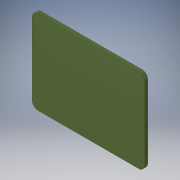
# Autodesk Inventor part: hanko_mat
Saved by Autodesk Inventor 2019 (Build 230136000, 136)
## iProperties
Created: 2020-10-19
Part Number: hanko_mat
Material: 一般
Document SubType Name: Modeling
Designer: Masato
Density: 1 g/cm^3
Appearance: 既定
Author: Masato
Autodesk Inventor part; units mm, degrees
ref_plane "YZ Plane" through (0, 0, 0) normal (1, 0, 0) x (0, 1, 0)
ref_plane "XZ Plane" through (0, 0, 0) normal (0, 1, 0) x (-1, 0, 0)
ref_plane "XY Plane" through (0, 0, 0) normal (0, 0, 1) x (1, 0, 0)
sketch "スケッチ1" plane through (0, 0, 0) normal (0, 0, 1) x (1, 0, 0)
  line L0 (-50, 37.5) -> (50, 37.5)
  line L1 (50, 37.5) -> (50, -37.5)
  line L2 (50, -37.5) -> (-50, -37.5)
  line L3 (-50, -37.5) -> (-50, 37.5)
  line L4 (-50, 37.5) -> (50, -37.5) construction
  line L5 (50, 37.5) -> (-50, -37.5) construction
  point P0 (0, 0)
  dimension "d0" = 100
  dimension "d1" = 75
  constraints: 12 end point, 2 midpoint, 2 parallel, 1 horizontal, 1 perpendicular
  measures "d0" distance of L1.end L2.end
  measures "d1" distance of L0.end L1.end
extrude "押し出し1" add sketch "スケッチ1" along normal blind 3
fillet "フィレット1" radius 5 4 edges at (-50, 37.5, 1.5) (50, 37.5, 1.5) (50, -37.5, 1.5) (-50, -37.5, 1.5)
